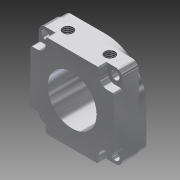
# Autodesk Inventor part: P60 Gearbox End Plate
Saved by Autodesk Inventor 2014 SP1 (Build 180222100, 222)
## iProperties
Created: 2012-01-14
Part Number: P60 Gearbox End Plate
Material: Aluminum-6061
Document SubType Name: Modeling
Designer: Moses
Density: 2.71 g/cm^3
Mass: 38.1981 g
Surface Area: 61.8488 cm^2
Volume: 14.0953 cm^3
Appearance: Aluminum - Polished
Author: Moses
Autodesk Inventor part; units mm, degrees
note: some values were not read from the file. Chosen so that the rebuilt part matches the saved one: sketch regions of "Extrusion2".
ref_plane "YZ Plane" through (0, 0, 0) normal (1, 0, 0) x (0, 1, 0)
ref_plane "XZ Plane" through (0, 0, 0) normal (0, 1, 0) x (-1, 0, 0)
ref_plane "XY Plane" through (0, 0, 0) normal (0, 0, 1) x (1, 0, 0)
sketch "Sketch1" plane through (0, 0, 0) normal (0, 0, 1) x (1, 0, 0)
  line L0 (0, 0) -> (38.1, 0)
  line L1 (38.1, 0) -> (38.1, 38.1)
  line L2 (38.1, 38.1) -> (0, 38.1)
  line L3 (0, 38.1) -> (0, 0)
  circle A0 centre (3.175, 34.925) radius 1.8796
  circle A1 centre (34.925, 34.925) radius 1.8796
  circle A2 centre (3.175, 3.175) radius 1.8796
  circle A3 centre (34.925, 3.175) radius 1.8796
  line L4 (0, 19.05) -> (19.05, 19.05) construction
  circle A4 centre (19.05, 19.05) radius 11.1125
  circle A5 centre (19.05, 19.05) radius 6.35
  line L5 (6.9596, 34.925) -> (6.9596, 38.1)
  line L6 (0, 31.1404) -> (3.175, 31.1404)
  arc A6 (3.175, 31.1404) -> (6.9596, 34.925) centre (3.175, 34.925) ccw
  line L7 (5.0546, 34.925) -> (6.9596, 34.925)
  line L8 (3.175, 6.9596) -> (0, 6.9596)
  line L9 (6.9596, 0) -> (6.9596, 3.175)
  arc A7 (6.9596, 3.175) -> (3.175, 6.9596) centre (3.175, 3.175) ccw
  line L10 (31.1404, 3.175) -> (31.1404, 0)
  line L11 (38.1, 6.9596) -> (34.925, 6.9596)
  arc A8 (34.925, 6.9596) -> (31.1404, 3.175) centre (34.925, 3.175) ccw
  line L12 (34.925, 31.1404) -> (38.1, 31.1404)
  line L13 (31.1404, 38.1) -> (31.1404, 34.925)
  arc A9 (31.1404, 34.925) -> (34.925, 31.1404) centre (34.925, 34.925) ccw
  line L14 (0, 6.9596) -> (0, 0)
  line L15 (0, 0) -> (6.9596, 0)
  line L16 (31.1404, 0) -> (38.1, 0)
  line L17 (38.1, 0) -> (38.1, 6.9596)
  line L18 (31.1404, 38.1) -> (38.1, 38.1)
  line L19 (38.1, 38.1) -> (38.1, 31.1404)
  dimension "d2" = 3.7592
  dimension "d0" = 38.1
  dimension "d1" = 38.1
  dimension "d5" = 31.75
  dimension "d8" = 31.75
  dimension "d11" = 3.175
  dimension "d12" = 3.175
  dimension "d13" = 19.05
  dimension "d14" = 22.225
  dimension "d15" = 12.7
  dimension "d16" = 3.175
  dimension "d17" = 3.175
  dimension "d18" = 1.905
  dimension "d24" = 360
  constraints: 40 end point, 9 centre point, 8 point on circle, 5 perpendicular, 3 coincident, 2 horizontal, 2 parallel, 2 point on line, 1 collinear, 1 horizontal alignment, 1 midpoint, 1 vertical, 41 other
  measures "d0" distance of L0.start L0.end
  measures "d1" distance of L0.end L1.end
  measures "d5" distance of point (3.175, 34.925) A1.centre
  measures "d8" distance of point (3.175, 34.925) A2.centre
  measures "d11" distance from line of L2 point (3.175, 34.925)
  measures "d12" distance from line of L3 point (3.175, 34.925)
  measures "d13" distance of L4.start L4.end
  measures "d14" diameter of A4
  measures "d15" diameter of A5
  measures "d16" distance of L5.start L5.end
  measures "d17" distance of L6.start L6.end
  measures "d18" distance of L7.start L5.start
extrude "Extrusion1" add sketch "Sketch1" along normal blind 3.81 contours L9 A7 L8 L3 L6 A6 L5 L2 L13 A9 L12 L1 L11 A8 L10 L0
extrude "Extrusion2" add sketch "Sketch1" against normal blind 11.43 contours L3 L8 A7 L9 L0 | L9 A7 L8 L3 L6 A6 L5 L2 L13 A9 L12 L1 L11 A8 L10 L0 | L10 A8 L11 L1 L0 | L3 L2 L5 A6 L6 | L12 A9 L13 L2 L1
fillet "Fillet1" radius 3.175 4 edges at (38.1, 38.1, -5.715) (38.1, 0, -5.715) (0, 38.1, -5.715) (0, 0, -5.715)
sketch "Sketch2" plane through (6.9596, 38.1, 3.81) normal (0, 1, 0) x (1, 0, 0)
  line L0 (12.0904, 7.62) -> (21.6154, 7.62)
  line L1 (12.0904, 7.62) -> (2.5654, 7.62)
  circle A0 centre (2.5654, 7.62) radius 2.3495
  circle A1 centre (21.6154, 7.62) radius 2.3495
  line L2 (0, 0) -> (24.1808, 0) projected
  line L3 (12.0904, 7.62) -> (12.0904, 0)
  point P0 (-6.9596, 3.81)
  dimension "d32" = 9.525
  dimension "d33" = 9.525
  dimension "d34" = 4.699
  dimension "d35" = 4.699
  dimension "d45" = 7.62
  constraints: 6 end point, 2 centre point, 2 coincident, 1 collinear, 1 horizontal, 1 midpoint, 1 vertical
  measures "d32" distance of L0.start L0.end
  measures "d33" distance of L0.start L1.end
  measures "d34" diameter of A0
  measures "d35" diameter of A1
  measures "d45" distance of L0.start L3.end
extrude "Extrusion3" cut sketch "Sketch2" against normal blind 3.81
sketch "Sketch3" plane through (6.9596, 0, 3.81) normal (0, -1, 0) x (1, 0, 0)
  line L0 (12.0904, -7.62) -> (21.6154, -7.62)
  line L1 (12.0904, -7.62) -> (2.5654, -7.62)
  circle A0 centre (2.5654, -7.62) radius 2.3495
  circle A1 centre (21.6154, -7.62) radius 2.3495
  line L2 (24.1808, 0) -> (0, 0) projected
  line L3 (12.0904, -7.62) -> (12.0904, 0)
  point P0 (-6.9596, -3.81)
  dimension "d39" = 9.525
  dimension "d40" = 9.525
  dimension "d41" = 4.699
  dimension "d42" = 4.699
  dimension "d46" = 7.62
  constraints: 6 end point, 2 centre point, 2 coincident, 1 collinear, 1 horizontal, 1 midpoint, 1 vertical
  measures "d39" distance of L0.start L0.end
  measures "d40" distance of L0.start L1.end
  measures "d41" diameter of A0
  measures "d42" diameter of A1
  measures "d46" distance of L0.start L3.end
extrude "Extrusion4" cut sketch "Sketch3" against normal blind 3.81
thread "Thread1" size "10-32 UNF" class "2B" standard "ANSI Unified Screw Threads" full length
thread "Thread2" size "10-32 UNF" class "2B" standard "ANSI Unified Screw Threads" full length
thread "Thread3" size "10-32 UNF" class "2B" standard "ANSI Unified Screw Threads" full length
thread "Thread4" size "10-32 UNF" class "2B" standard "ANSI Unified Screw Threads" full length
fillet "Fillet2" radius 1 8 edges at (38.1, 31.1404, 1.905) (31.1404, 38.1, 1.905) (31.1404, 0, 1.905) (38.1, 6.9596, 1.905) (6.9596, 38.1, 1.905) (0, 31.1404, 1.905) (0, 6.9596, 1.905) (6.9596, 0, 1.905)
sketch "Sketch4" plane through (0, 0, -11.43) normal (0, 0, -1) x (-1, 0, 0)
  arc A0 (-3.175, 0) -> (0, 3.175) centre (-3.175, 3.175) ccw projected
  line L0 (0, 34.925) -> (0, 3.175) projected
  arc A1 (0, 34.925) -> (-3.175, 38.1) centre (-3.175, 34.925) ccw projected
  line L1 (-34.925, 38.1) -> (-3.175, 38.1) projected
  arc A2 (-34.925, 38.1) -> (-38.1, 34.925) centre (-34.925, 34.925) ccw projected
  line L2 (-38.1, 3.175) -> (-38.1, 34.925) projected
  arc A3 (-38.1, 3.175) -> (-34.925, 0) centre (-34.925, 3.175) ccw projected
  line L3 (-3.175, 0) -> (-34.925, 0) projected
  circle A4 centre (-3.175, 34.925) radius 1.8796 projected
  circle A5 centre (-19.05, 19.05) radius 11.1125 projected
  circle A6 centre (-34.925, 3.175) radius 1.8796 projected
  arc A7 (-0.5, 34.925) -> (-3.175, 37.6) centre (-3.175, 34.925) ccw
  line L4 (-0.5, 34.925) -> (-0.5, 3.175)
  arc A8 (-3.175, 0.5) -> (-0.5, 3.175) centre (-3.175, 3.175) ccw
  line L5 (-3.175, 0.5) -> (-34.925, 0.5)
  arc A9 (-37.6, 3.175) -> (-34.925, 0.5) centre (-34.925, 3.175) ccw
  line L6 (-37.6, 3.175) -> (-37.6, 34.925)
  arc A10 (-34.925, 37.6) -> (-37.6, 34.925) centre (-34.925, 34.925) ccw
  line L7 (-34.925, 37.6) -> (-3.175, 37.6)
  circle A11 centre (-19.05, 19.05) radius 18.415 construction
  line L8 (-25.187, 1.6877) -> (-36.4123, 12.913) construction
  line L9 (-1.6877, 25.187) -> (-12.913, 36.4123) construction
  line L10 (-28.0467, 2.9823) -> (-35.1177, 10.0533) construction
  line L11 (-2.9823, 28.0467) -> (-10.0533, 35.1177) construction
  circle A12 centre (-35.1177, 10.0533) radius 1.1067
  circle A13 centre (-28.0467, 2.9823) radius 1.1067
  circle A14 centre (-10.0533, 35.1177) radius 1.1067
  circle A15 centre (-2.9823, 28.0467) radius 1.1067
  circle A16 centre (-19.05, 19.05) radius 14.75
  arc A17 (-19.05, 0.5) -> (-0.5, 19.05) centre (-19.05, 19.05) ccw
  arc A18 (-19.05, 37.6) -> (-37.6, 19.05) centre (-19.05, 19.05) ccw
  point P0 (0, 0)
  dimension "d59" = 36.83
  dimension "d56" = 0.5
  dimension "d60" = 15.875
  dimension "d64" = 10
  dimension "d65" = 29.5
  dimension "d68" = 45
  constraints: 16 end point, 12 point on circle, 11 centre point, 6 coincident, 6 tangent, 5 parallel, 4 midpoint, 17 other
  measures "d56" distance between parallel lines of L1 L7
  measures "d60" distance of L8.start L8.end
  measures "d64" distance of L10.start L10.end
  measures "d65" diameter of A16
  measures "d68" angle of L5 L10
extrude "Extrusion5" cut sketch "Sketch4" against normal blind 4 contours L3 A3 L2 A2 L1 A1 L0 A0 | A5 | L4 A8 L5 A17 | A18 L6 A10 L7 | A12 | A13 | A14 | A15
extrude "Extrusion6" add sketch "Sketch4" along normal blind 1 contours A16
equation "\"d16\" = d11"
equation "\"d17\" = d11"
body "Solid1"
